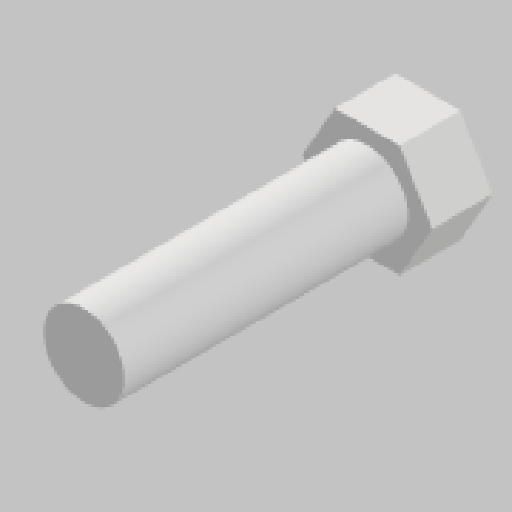
# Autodesk Inventor part: Perno
Saved by Autodesk Inventor 2024 (Build 280153000, 153)
## iProperties
Created: 2023-09-27
Part Number: Perno
Material: Generic
Document SubType Name: Modeling
Designer: ARViau
Density: 1 g/cm^3
Appearance: Default
Author: ARViau
Autodesk Inventor part; units mm, degrees
ref_plane "YZ Plane" through (0, 0, 0) normal (1, 0, 0) x (0, 1, 0)
ref_plane "XZ Plane" through (0, 0, 0) normal (0, 1, 0) x (-1, 0, 0)
ref_plane "XY Plane" through (0, 0, 0) normal (0, 0, 1) x (1, 0, 0)
sketch "Sketch1" plane through (0, 0, 0) normal (0, 0, 1) x (1, 0, 0)
  circle A0 centre (0, 0) radius 10.16
  dimension "d0" = 20.32
  constraints: 1 centre point, 1 coincident
  measures "d0" diameter of A0
extrude "Extrusion1" add sketch "Sketch1" against normal blind 9.525
sketch "Sketch2" plane through (0, 0, -9.525) normal (0, 0, -1) x (-1, 0, 0)
  circle A0 centre (0, 0) radius 10.16 projected
  line L0 (-10.16, 0) -> (-5.08, 8.7988)
  line L1 (-5.08, 8.7988) -> (5.08, 8.7988)
  line L2 (5.08, 8.7988) -> (10.16, 0)
  line L3 (10.16, 0) -> (5.08, -8.7988)
  line L4 (5.08, -8.7988) -> (-5.08, -8.7988)
  line L5 (-5.08, -8.7988) -> (-10.16, 0)
  point P0 (10.16, 0)
  point P1 (10.16, 0)
  point P2 (5.08, 8.7988)
  point P3 (5.08, 8.7988)
  point P4 (-5.08, 8.7988)
  point P5 (-5.08, 8.7988)
  constraints: 12 end point, 1 coincident, 1 horizontal alignment, 15 other
extrude "Extrusion2" cut sketch "Sketch2" against normal blind 9.525 contours L2 A0 | A0 L3 | L1 A0 | A0 L4 | L0 A0 | A0 L5
sketch "Sketch3" plane through (0, 0, 0) normal (0, 0, 1) x (1, 0, 0)
  circle A0 centre (0, 0) radius 6.35
  dimension "d5" = 12.7
  constraints: 1 centre point, 1 coincident
  measures "d5" diameter of A0
extrude "Extrusion3" add sketch "Sketch3" along normal blind 44.45
sketch "Sketch4" plane through (0, 0, 44.45) normal (0, 0, 1) x (1, 0, 0)
  circle A0 centre (0, 0) radius 6.35 construction
  circle A1 centre (0, 0) radius 4.7625
  dimension "d8" = 9.525
  constraints: 1 centre point, 1 coincident
  measures "d8" diameter of A1
extrude "Extrusion4" add sketch "Sketch4" along normal blind 12.7
chamfer "Chamfer1" distance 1.27 angle 45 1 edges at (-4.7625, 0, 57.15)
body "Solid1"
